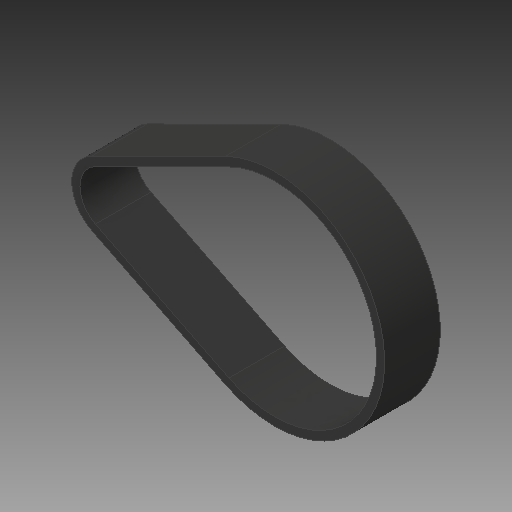
# Autodesk Inventor part: Belt
Saved by Autodesk Inventor 2019.3 (Build 233278000, 278)
## iProperties
Created: 2019-03-02
Part Number: Belt
Material: Rubber, Silicone
Document SubType Name: Modeling
Designer: Petar
Density: 1.25 g/cm^3
Appearance: Rubber - Black
Mass: 9.72075 g
Surface Area: 81.0652 cm^2
Volume: 7.7766 cm^3
Author: Petar
Autodesk Inventor part; units mm, degrees
ref_plane "YZ Plane" through (0, 0, 0) normal (1, 0, 0) x (0, 1, 0)
ref_plane "XZ Plane" through (0, 0, 0) normal (0, 1, 0) x (-1, 0, 0)
ref_plane "XY Plane" through (0, 0, 0) normal (0, 0, 1) x (1, 0, 0)
sketch "Sketch1" plane through (0, 0, 0) normal (0, 0, 1) x (1, 0, 0)
  circle A0 centre (0, 0) radius 8.217 construction
  line L0 (0, 0) -> (45, 0) construction
  arc A1 (-3.3497, 6.7294) -> (-3.3497, -6.7294) centre (0, 0) ccw
  arc A2 (9.717, 0) -> (2.1626, 9.4733) centre (0, 0) ccw construction
  circle A3 centre (45, 0) radius 28.27 construction
  arc A4 (32.7142, -24.6812) -> (32.7142, 24.6812) centre (45, 0) ccw
  arc A5 (15.23, 0) -> (22.6595, -19.6762) centre (45, 0) ccw construction
  line L1 (-4.3301, 8.6989) -> (31.7338, 26.6507)
  line L2 (-4.3301, -8.6989) -> (31.7338, -26.6507)
  line L3 (-3.3497, 6.7294) -> (32.7142, 24.6812)
  line L4 (-3.3497, -6.7294) -> (32.7142, -24.6812)
  arc A6 (17.43, 0) -> (32.7142, -24.6812) centre (45, 0) ccw construction
  arc A7 (32.7142, 24.6812) -> (17.43, 0) centre (45, 0) ccw construction
  arc A8 (7.517, 0) -> (-3.3497, 6.7294) centre (0, 0) ccw construction
  arc A9 (-3.3497, -6.7294) -> (7.517, 0) centre (0, 0) ccw construction
  arc A10 (2.1626, -9.4733) -> (9.717, 0) centre (0, 0) ccw construction
  arc A11 (2.1626, 9.4733) -> (-4.3301, 8.6989) centre (0, 0) ccw construction
  arc A12 (22.6595, 19.6762) -> (15.23, 0) centre (45, 0) ccw construction
  arc A13 (22.6595, -19.6762) -> (31.7338, -26.6507) centre (45, 0) ccw construction
  arc A14 (-4.3301, 8.6989) -> (-4.3301, -8.6989) centre (0, 0) ccw
  arc A15 (-4.3301, -8.6989) -> (2.1626, -9.4733) centre (0, 0) ccw construction
  arc A16 (31.7338, 26.6507) -> (22.6595, 19.6762) centre (45, 0) ccw construction
  arc A17 (31.7338, -26.6507) -> (31.7338, 26.6507) centre (45, 0) ccw
  dimension "d0" = 16.434
  dimension "d1" = 45
  dimension "d3" = 1.5
  dimension "d4" = 56.54
  dimension "d5" = 0.7
  dimension "d6" = 0.7
  dimension "d7" = 1.5
  constraints: 34 point on circle, 18 centre point, 12 tangent, 10 end point, 8 point on line, 6 coincident, 4 symmetric about line, 1 horizontal
  measures "d0" diameter of A0
  measures "d1" distance of L0.start L0.end
  measures "d3" radial gap between concentric circles of A2 A0
  measures "d4" diameter of A3
  measures "d5" radial gap between concentric circles of A1 A0
  measures "d6" radial gap between concentric circles of A4 A3
  measures "d7" radial gap between concentric circles of A3 A5
extrude "Extrusion1" add sketch "Sketch1" along normal blind 15
body "Solid1"
